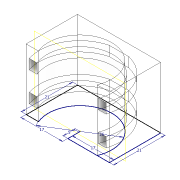
# Autodesk Inventor part: abrazadera_smps
Saved by Autodesk Inventor 2018 (Build 220112000, 112)
## iProperties
Created: 2018-08-02
Part Number: abrazadera_smps
Material: Generic
Document SubType Name: Sheet Metal
Designer: Bardo91
Density: 1 g/cm^3
Sheet Metal Rule: Default_mm
Appearance: Default
Author: Bardo91
Autodesk Inventor part; units mm, degrees
ref_plane "YZ Plane" through (0, 0, 0) normal (1, 0, 0) x (0, 1, 0)
ref_plane "XZ Plane" through (0, 0, 0) normal (0, 1, 0) x (-1, 0, 0)
ref_plane "XY Plane" through (0, 0, 0) normal (0, 0, 1) x (1, 0, 0)
sketch "Sketch1" plane through (0, 0, 0) normal (0, 0, 1) x (1, 0, 0)
  arc A0 (12, -5) -> (-12, -5) centre (0, 0) ccw
  line L0 (0, 0) -> (0, -5)
  line L1 (-12, -5) -> (-17, -5)
  line L2 (-17, -5) -> (-17, 16)
  line L3 (0, -5) -> (17, -5)
  line L4 (17, -5) -> (17, 16)
  line L5 (17, 16) -> (-17, 16)
  dimension "d0" = 26
  dimension "d1" = 5
  dimension "d2" = 17
  dimension "d3" = 21
  dimension "d4" = 17
  dimension "d5" = 21
  constraints: 12 end point, 3 perpendicular, 2 point on circle, 1 centre point, 1 coincident, 1 horizontal, 1 point on line, 1 vertical
  measures "d0" diameter of A0
  measures "d1" distance of L0.start L0.end
  measures "d2" distance of L0.end L1.end
  measures "d3" distance of L1.end L2.end
  measures "d4" distance of L0.end L3.end
  measures "d5" distance of L3.end L4.end
extrude "Extrusion1" add sketch "Sketch1" along normal blind 25
ref_plane "Work Plane1" through (0, 0, 0) normal (0, -1, 0) x (1, 0, 0)
sketch "Sketch2" plane through (0, 0, 0) normal (0, -1, 0) x (1, 0, 0)
  line L0 (0, 0) -> (0, 25)
  line L1 (-13, 25) -> (13, 25) projected
  line L2 (0, 12.5) -> (-13, 12.5)
  line L3 (-13, 12.5) -> (-15, 12.5)
  line L4 (-15, 12.5) -> (-15, 16.5)
  line L5 (-15, 16.5) -> (-13.5, 16.5)
  line L6 (-13.5, 16.5) -> (-13.5, 20.5)
  line L7 (-13.5, 20.5) -> (-16.5, 20.5)
  line L8 (-16.5, 20.5) -> (-16.5, 16.5)
  line L9 (-16.5, 16.5) -> (-15, 16.5)
  line L10 (-15, 12.5) -> (-15, 8.5)
  line L11 (-15, 8.5) -> (-13.5, 8.5)
  line L12 (-13.5, 8.5) -> (-13.5, 4.5)
  line L13 (-13.5, 4.5) -> (-16.5, 4.5)
  line L14 (-16.5, 4.5) -> (-16.5, 8.5)
  line L15 (-16.5, 8.5) -> (-15, 8.5)
  line L16 (13, 12.5) -> (15, 12.5)
  line L17 (15, 12.5) -> (15, 16.5)
  line L18 (15, 16.5) -> (13.5, 16.5)
  line L19 (13.5, 16.5) -> (13.5, 20.5)
  line L20 (13.5, 20.5) -> (16.5, 20.5)
  line L21 (16.5, 20.5) -> (16.5, 16.5)
  line L22 (16.5, 16.5) -> (15, 16.5)
  line L23 (15, 12.5) -> (15, 8.5)
  line L24 (15, 8.5) -> (13.5, 8.5)
  line L25 (13.5, 8.5) -> (13.5, 4.5)
  line L26 (13.5, 4.5) -> (16.5, 4.5)
  line L27 (16.5, 4.5) -> (16.5, 8.5)
  line L28 (16.5, 8.5) -> (15, 8.5)
  point P0 (-12, 25)
  point P1 (12, 25)
  dimension "d8" = 2
  dimension "d9" = 4
  dimension "d10" = 1.5
  dimension "d11" = 4
  dimension "d12" = 3
  dimension "d13" = 4
  constraints: 56 end point, 17 symmetric about line, 5 point on line, 4 perpendicular, 2 midpoint, 1 horizontal
  measures "d8" distance of L2.end L3.end
  measures "d9" distance of L3.end L4.end
  measures "d10" distance of L4.end L5.end
  measures "d11" distance of L5.end L6.end
  measures "d12" distance of L6.end L7.end
  measures "d13" distance of L7.end L8.end
revolve "Revolution1" cut sketch "Sketch2" angle 180 about axis through (0, 0, 0) along (0, 0, -1)
equation "\"BendRadius\" = Thickness"
equation "\"BendReliefWidth\" = Thickness"
equation "\"BendReliefDepth\" = 0.5 * Thickness"
equation "\"CornerReliefSize\" = 4 * Thickness"
equation "\"MinimumRemnant\" = 2 * Thickness"
equation "\"TransitionRadius\" = BendRadius"
equation "\"JacobiRadiusSize\" = BendRadius"
equation "\"GapSize\" = Thickness"
equation "\"Thickness\" = 0.5"
body "Solid1"
